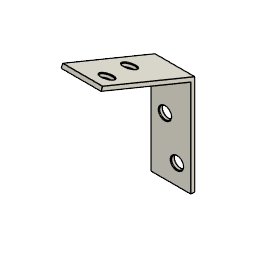
top_panel_bracket (Autodesk Fusion 360 design; units mm, degrees)
Autodesk Fusion 360 part; units mm, degrees
sketch "Sketch1" plane through (0, 0, 0) normal (1, 0, 0) x (0, 1, 0)
  line L0 (0, 0) -> (0, 50)
  line L1 (0, 50) -> (-46.2605, 68.9728)
  line L2 (-46.2605, 68.9728) -> (-47.0194, 67.1224)
  line L3 (-47.0194, 67.1224) -> (-2, 48.6586)
  line L4 (-2, 48.6586) -> (-2, 0)
  line L5 (-2, 0) -> (0, 0)
  dimension "d1" = 2
  dimension "d2" = 2
  dimension "d3" = 50
  dimension "d4" = 50
  dimension "d27" = 112.3
  constraint coincident L0.start L5.end
  constraint vertical L0
  constraint perpendicular L1 L2
  constraint perpendicular L2 L3
  constraint vertical L4
  constraint perpendicular L0 L5
  measures "d1" distance of L1.end L2.end
  measures "d2" distance of L4.end L0.start
  measures "d3" distance of L0.start L0.end
  measures "d4" distance of L0.end L1.end
  measures "d27" angle of L3 L4
extrude "Extrude1" add sketch "Sketch1" against normal blind 20
sketch "Sketch2" plane through (0, -2, 0) normal (0, -1, 0) x (1, 0, 0)
  line L0 (0, 0) -> (0, 48.6586)
  line L1 (0, 48.6586) -> (-20, 48.6586)
  line L2 (-20, 48.6586) -> (-20, 0)
  line L3 (-20, 0) -> (0, 0)
  circle A0 centre (-13, 28.6586) radius 3
  circle A1 centre (-7, 10) radius 3
  point P0 (0, 50)
  dimension "d7" = 10
  dimension "d8" = 20
  dimension "d10" = 18.6586
  dimension "d11" = 7
  dimension "d12" = 7
  dimension "d13" = 6
  dimension "d14" = 6
  measures "d7" distance of L3 A1.centre
  measures "d8" distance of L1 A0.centre
  measures "d10" vertical distance of A0.centre A1.centre
  measures "d11" distance of L2 A0.centre
  measures "d12" distance of L0 A1.centre
  measures "d13" diameter of A0
  measures "d14" diameter of A1
sketch "Sketch3" plane through (0, 16.7949, 40.9502) normal (0, -0.379456, -0.92521) x (1, 0, 0)
  line L0 (0, 20.3142) -> (0, 68.9728)
  line L1 (0, 68.9728) -> (-20, 68.9728)
  line L2 (-20, 68.9728) -> (-20, 20.3142)
  line L3 (-20, 20.3142) -> (0, 20.3142)
  circle A0 centre (-7, 58.9728) radius 3
  circle A1 centre (-13, 40.3142) radius 3
  line L4 (0, 20.3142) -> (-20, 20.3142)
  dimension "d15" = 6
  dimension "d16" = 6
  dimension "d17" = 7
  dimension "d18" = 7
  dimension "d19" = 10
  dimension "d20" = 20
  dimension "d28" = 18.6586
  measures "d15" diameter of A0
  measures "d16" diameter of A1
  measures "d17" distance of L0 A0.centre
  measures "d18" distance of L2 A1.centre
  measures "d19" distance of L1 A0.centre
  measures "d20" distance of A1.centre L4
  measures "d28" vertical distance of A0.centre A1.centre
extrude "Extrude2" cut sketch "Sketch3" against normal blind 2 contours A0 | A1
extrude "Extrude3" cut sketch "Sketch2" against normal blind 2 contours A0 | A1
fillet "Fillet1" radius 0.3 8 edges at (-9.797, -38.771, 63.7395) (-15.797, -21.5079, 56.6594) (-15.797, -2, 29.7434) (-9.797, -2, 11.0848) (-9.797, 0, 8.9152) (-15.797, 0, 27.5737) (-9.797, -36.0047, 64.7666) (-15.797, -18.7416, 57.6865)
named bodies: "Top Panel and Back Panel Bracket"
